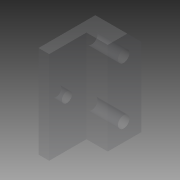
# Autodesk Inventor part: switchlock2
Saved by Autodesk Inventor 2015 (Build 190159000, 159)
## iProperties
Created: 2020-08-08
Part Number: switchlock2
Material: 일반
Document SubType Name: Modeling
Designer: penta
Density: 1 g/cm^3
Appearance: 기본값
Author: penta
Autodesk Inventor part; units mm, degrees
ref_plane "YZ Plane" through (0, 0, 0) normal (1, 0, 0) x (0, 1, 0)
ref_plane "XZ Plane" through (0, 0, 0) normal (0, 1, 0) x (-1, 0, 0)
ref_plane "XY Plane" through (0, 0, 0) normal (0, 0, 1) x (1, 0, 0)
sketch "스케치1" plane through (0, 0, 0) normal (0, 1, 0) x (-1, 0, 0)
  line L0 (0, 0) -> (-6, 0)
  line L1 (-6, 0) -> (-6, -26)
  line L2 (-6, -26) -> (0, -26)
  line L3 (0, -26) -> (0, 0)
  dimension "d0" = 6
  dimension "d1" = 26
  constraints: 8 end point, 2 parallel, 1 horizontal, 1 perpendicular
  measures "d0" distance of L2.end L1.end
  measures "d1" distance of L1.end L0.end
extrude "돌출1" add sketch "스케치1" along normal blind 10
sketch "스케치2" plane through (0, 10, 0) normal (0, 1, 0) x (1, 0, 0)
  line L0 (6, 26) -> (0, 26)
  line L1 (-3, 26) -> (-3, 0)
  line L2 (-3, 0) -> (0, 0)
  line L3 (6, 0) -> (6, 26)
  line L4 (0, 0) -> (0, 26)
  line L5 (0, 26) -> (-3, 26)
  line L6 (0, 0) -> (6, 0)
  dimension "d4" = 9
  constraints: 14 end point, 5 parallel, 4 perpendicular, 2 horizontal
  measures "d4" distance of L3.start L1.end
extrude "돌출2" add sketch "스케치2" against normal blind 20 contours L4 L2 L1 L5
hole "구멍1" at (-3, 5, -21) direction (1, 0, 0) diameter 3.25 end through all
hole "구멍2" at (-3, 5, -5) direction (1, 0, 0) diameter 3.25 end through all
hole "구멍3" at (-3, -5, -13) direction (1, 0, 0) diameter 2.85 end through all
thicken "두껍게 하기1" operation add thickness 0.5 both sides no extend neighbours yes toward (0, 1, 0) faces at (4, 0, -8.6667)
chamfer "모따기1" distance 4 angle 45 1 edges at (1.5, 10, 0)
